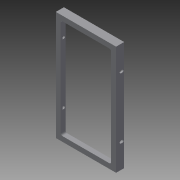
# Autodesk Inventor part: RahmenV04_TOP
Saved by Autodesk Inventor 2015 (Build 190159000, 159)
## iProperties
Created: 2016-07-21
Part Number: RahmenV04_TOP
Material: Generic
Document SubType Name: Modeling
Designer: spichelh
Density: 1 g/cm^3
Appearance: Default
Author: spichelh
Autodesk Inventor part; units mm, degrees
ref_plane "YZ Plane" through (0, 0, 0) normal (1, 0, 0) x (0, 1, 0)
ref_plane "XZ Plane" through (0, 0, 0) normal (0, 1, 0) x (-1, 0, 0)
ref_plane "XY Plane" through (0, 0, 0) normal (0, 0, 1) x (1, 0, 0)
sketch "Sketch1" plane through (0, 0, 0) normal (0, 1, 0) x (-1, 0, 0)
  line L0 (33.575, 60.88) -> (-33.575, 60.88)
  line L1 (-33.575, 60.88) -> (-33.575, -60.88)
  line L2 (-33.575, -60.88) -> (33.575, -60.88)
  line L3 (33.575, -60.88) -> (33.575, 60.88)
  line L4 (21.765, 52.07) -> (27.765, 52.07) construction
  line L5 (0, 0) -> (-80.4548, 0) construction
  line L6 (0, 0) -> (0, 46.6746) construction
  line L7 (28.575, 55.88) -> (-28.575, 55.88) construction
  line L8 (-28.575, 55.88) -> (-28.575, -55.88) construction
  line L9 (-28.575, -55.88) -> (28.575, -55.88) construction
  line L10 (28.575, -55.88) -> (28.575, 55.88) construction
  circle A0 centre (24.765, 52.07) radius 1.5 construction
  circle A1 centre (-24.765, 52.07) radius 1.5 construction
  circle A2 centre (24.765, -41.91) radius 3.8303 construction
  circle A3 centre (-24.765, -41.91) radius 3.8303 construction
  line L11 (26.075, 55.38) -> (-26.075, 55.38)
  line L12 (-26.075, -55.38) -> (26.075, -55.38)
  line L13 (28.575, 55.88) -> (-28.575, -55.88) construction
  line L14 (28.575, -55.88) -> (-28.575, 55.88) construction
  line L15 (28.075, -53.38) -> (28.075, 53.38)
  arc A4 (26.075, -55.38) -> (28.075, -53.38) centre (26.075, -53.38) ccw
  arc A5 (-28.075, -53.38) -> (-26.075, -55.38) centre (-26.075, -53.38) ccw
  line L16 (-28.075, 53.38) -> (-28.075, -53.38)
  arc A6 (28.075, 53.38) -> (26.075, 55.38) centre (26.075, 53.38) ccw
  arc A7 (-26.075, 55.38) -> (-28.075, 53.38) centre (-26.075, 53.38) ccw
  point P0 (28.075, 55.38)
  point P1 (-28.075, 55.38)
  dimension "d77" = 57.15
  dimension "d78" = 3.81
  dimension "d79" = 3.81
  dimension "d80" = 3.81
  dimension "d81" = 3.81
  dimension "d82" = 3
  dimension "d85" = 111.76
  dimension "d88" = 3.81
  dimension "d100" = 0.5
  dimension "d101" = 5
  dimension "d104" = 0.5
  dimension "d107" = 5
  dimension "d109" = 5
  dimension "d115" = 0.5
  dimension "d122" = 5
  dimension "d123" = 2
  dimension "d129" = 0.5
  dimension "d130" = 2
  constraints: 35 end point, 8 centre point, 8 point on circle, 8 tangent, 6 parallel, 5 horizontal, 4 point on line, 3 perpendicular, 2 equal radius, 2 midpoint, 1 coincident, 1 symmetric about line, 1 vertical, 1 other
  measures "d77" distance of L7.start L7.end
  measures "d78" distance from line of L8 A1.centre
  measures "d79" distance from line of L7 A1.centre
  measures "d80" distance from line of L7 A0.centre
  measures "d81" distance from line of L10 A0.centre
  measures "d82" diameter of A0
  measures "d85" distance of L9.end L7.start
  measures "d88" distance from line of L10 A2.centre
  measures "d100" distance between parallel lines of L7 L11
  measures "d101" distance between parallel lines of L0 L7
  measures "d104" distance between parallel lines of L9 L12
  measures "d107" distance between parallel lines of L2 L9
  measures "d109" distance between parallel lines of L3 L10
  measures "d115" distance between parallel lines of L10 L15
  measures "d122" distance between parallel lines of L8 L1
  measures "d123" radius of A4
  measures "d129" distance between parallel lines of L8 L16
  measures "d130" radius of A6
extrude "Extrusion1" add sketch "Sketch1" along normal blind 9
sketch "Sketch5" plane through (0, 9, 0) normal (0, 1, 0) x (1, 0, 0)
  line L0 (-29.675, 58.98) -> (29.675, 58.98)
  line L1 (31.675, 56.98) -> (31.675, -56.98)
  line L2 (29.675, -58.98) -> (-29.675, -58.98)
  line L3 (-31.675, -56.98) -> (-31.675, 56.98)
  line L4 (33.575, 60.88) -> (-33.575, 60.88) projected
  arc A0 (-29.675, 58.98) -> (-31.675, 56.98) centre (-29.675, 56.98) ccw
  arc A1 (31.675, 56.98) -> (29.675, 58.98) centre (29.675, 56.98) ccw
  arc A2 (29.675, -58.98) -> (31.675, -56.98) centre (29.675, -56.98) ccw
  arc A3 (-31.675, -56.98) -> (-29.675, -58.98) centre (-29.675, -56.98) ccw
  line L5 (-33.575, 60.88) -> (-33.575, -60.88) projected
  line L6 (33.575, -60.88) -> (33.575, 60.88) projected
  line L7 (-33.575, -60.88) -> (33.575, -60.88) projected
  point P0 (0, 0)
  point P1 (-31.675, 58.98)
  point P2 (31.675, -58.98)
  point P3 (31.675, 58.98)
  point P4 (-31.675, -58.98)
  dimension "d131" = 1.9
  dimension "d134" = 2
  dimension "d135" = 1.9
  dimension "d136" = 1.9
  dimension "d137" = 1.9
  dimension "d138" = 63.35
  constraints: 8 end point, 8 point on circle, 8 point on line, 8 tangent, 4 centre point, 3 equal radius, 2 parallel, 1 horizontal, 1 perpendicular
  measures "d131" distance between parallel lines of L0 L4
  measures "d134" radius of A0
  measures "d135" distance between parallel lines of L5 L3
  measures "d136" distance between parallel lines of L6 L1
  measures "d137" distance between parallel lines of L7 L2
  measures "d138" distance between parallel lines of L3 L1
extrude "Extrusion5" cut sketch "Sketch5" against normal blind 7 contours L0 A1 L1 A2 L2 A3 L3 A0
sketch "Sketch6" plane through (-33.575, 0, -60.88) normal (-1, 0, 0) x (0, 0, 1)
  circle A0 centre (94.76, 7) radius 1.5
  circle A1 centre (27, 5.5) radius 1.5
  line L0 (0, 0) -> (121.76, 0) projected
  line L1 (121.76, 0) -> (121.76, 9) projected
  line L2 (0, 0) -> (0, 9) projected
  circle A2 centre (94.76, 5.5) radius 1.5
  line L3 (94.76, 7) -> (94.76, 5.5) construction
  line L4 (93.26, 7) -> (93.26, 5.5)
  line L5 (96.26, 7) -> (96.26, 5.5)
  circle A3 centre (27, 7) radius 1.5
  line L6 (27, 5.5) -> (27, 7) construction
  line L7 (28.5, 5.5) -> (28.5, 7)
  line L8 (25.5, 5.5) -> (25.5, 7)
  point P0 (60.88, 0)
  point P1 (28.5, 7)
  point P2 (25.5, 7)
  dimension "d139" = 3
  dimension "d140" = 7
  dimension "d141" = 5.5
  dimension "d142" = 27
  dimension "d143" = 27
  dimension "d146" = 3
  dimension "d147" = 3
  dimension "d148" = 1.5
  dimension "d149" = 1.5
  constraints: 12 end point, 12 point on circle, 4 centre point, 4 tangent, 4 vertical, 1 equal radius
  measures "d139" diameter of A0
  measures "d140" distance from line of L0 L3.start
  measures "d141" distance from line of L0 L6.start
  measures "d142" distance from line of L1 L3.start
  measures "d143" distance from line of L2 L6.start
  measures "d146" diameter of A2
  measures "d147" diameter of A3
  measures "d148" distance of L8.start L8.end
  measures "d149" distance of L7.start L7.end
extrude "Extrusion6" cut sketch "Sketch6" against normal blind 70
body "Solid1"
